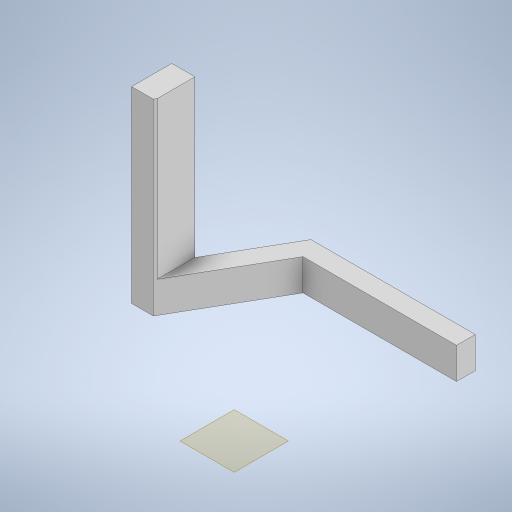
# Autodesk Inventor part: HexMidPiece
Saved by Autodesk Inventor 2024.2 (Build 282272000, 272)
## iProperties
Created: 2024-02-28
Part Number: HexMidPiece
Material: Generic
Document SubType Name: Modeling
Designer: Jared
Density: 1 g/cm^3
Appearance: Default
Author: Jared
Autodesk Inventor part; units mm, degrees
ref_plane "YZ Plane" through (0, 0, 0) normal (1, 0, 0) x (0, 1, 0)
ref_plane "XZ Plane" through (0, 0, 0) normal (0, 1, 0) x (-1, 0, 0)
ref_plane "XY Plane" through (0, 0, 0) normal (0, 0, 1) x (1, 0, 0)
ref_plane "Work Plane1" through (0, 12.7, 0) normal (0, 1, 0) x (1, 0, 0)
sketch "Sketch3" plane through (0, 12.7, 0) normal (0, 1, 0) x (1, 0, 0)
  line L0 (-42.4994, 73.6111) -> (4.3994, 73.6111)
  line L1 (-38.1, 65.9911) -> (-42.4994, 73.6111)
  line L2 (-38.1, 65.9911) -> (-60.325, 27.4963)
  line L3 (-60.325, 27.4963) -> (-69.1238, 27.4963)
  line L4 (0, 65.9911) -> (-38.1, 65.9911)
  line L5 (-42.4994, 73.6111) -> (-59.7198, 43.7846)
  line L6 (-59.7198, 43.7846) -> (-50.9209, 43.7846)
  line L7 (-42.4994, 73.6111) -> (-69.1238, 27.4963)
  line L8 (-42.4994, 73.6111) -> (24.1756, 73.6111)
  line L9 (24.1756, 73.6111) -> (24.1756, 65.9911)
  line L10 (24.1756, 65.9911) -> (0, 65.9911)
  line L11 (-69.1238, 27.4963) -> (-69.1238, 43.7846)
  line L12 (-69.1238, 43.7846) -> (-59.7198, 43.7846)
  line L13 (-59.7198, 43.7846) -> (-59.7198, 27.4963)
  point P0 (4.3994, 73.6111)
  point P1 (-59.7198, 28.5446)
  dimension "d49" = 46.8988
  dimension "d54" = 8.7988
  dimension "d61" = 120
  dimension "d64" = 60
  dimension "d65" = 38.1
  dimension "d75" = 66.675
  dimension "d88" = 44.45
  constraints: 28 end point, 4 horizontal, 3 perpendicular, 3 point on line, 2 collinear, 1 equal length, 1 vertical
  measures "d49" distance of L0.start L0.end
  measures "d54" distance of L1.start L1.end
  measures "d61" angle of L4 L2
  measures "d64" angle of L0 L1
  measures "d65" distance of L4.start L4.end
  measures "d75" distance of L1.end L8.end
  measures "d88" distance of L1.start L2.end
extrude "Extrusion12" add sketch "Sketch3" along normal blind 76.2 contours L13 L2 L3 L7 | L7 L11 L12
extrude "Extrusion13" add sketch "Sketch3" along normal blind 12.7 contours L0 L8 L9 L10 L4 L1 | L1 L2 L6 L5 | L6 L2 L13
body "Solid6"
